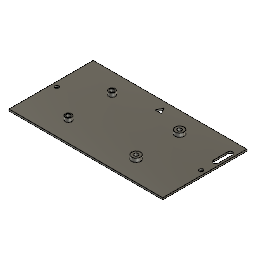
smmb_inner-middle (Autodesk Fusion 360 design; units mm, degrees)
Autodesk Fusion 360 part; units mm, degrees
sketch "Sketch1" plane through (0, 0, 0) normal (0, 0, 1) x (1, 0, 0)
  line L0 (0, 0) -> (127.5, 0)
  line L1 (127.5, 0) -> (127.5, 70)
  line L2 (127.5, 70) -> (0, 70)
  line L3 (0, 70) -> (0, 0)
  circle A0 centre (4, 35.763) radius 1.55
  line L4 (63.75, 0) -> (63.75, 70) construction
  circle A1 centre (123.5, 35.763) radius 1.55
  line L5 (66.25, 60) -> (61.25, 60)
  line L6 (61.25, 60) -> (61.25, 65)
  line L7 (61.25, 65) -> (66.25, 65)
  line L8 (66.25, 65) -> (66.25, 60)
  line L9 (66.25, 60) -> (61.25, 65) construction
  line L10 (61.25, 60) -> (66.25, 65) construction
  line L11 (63.75, 65) -> (61.25, 60)
  line L12 (63.75, 65) -> (66.25, 60)
  point P0 (63.75, 62.5)
  dimension "d1" = 127.5
  dimension "d2" = 70
  dimension "d3" = 3.1
  dimension "d4" = 35.763
  dimension "d5" = 4
  dimension "d8" = 5
  dimension "d9" = 5
  dimension "d12" = 5
  constraint horizontal L0
  constraint vertical L1
  constraint horizontal L2
  constraint vertical L3
  constraint coincident L0.start L3.end
  constraint midpoint L0 L4.start
  constraint midpoint L2 L4.end
  constraint symmetric A0 L4 A1
  constraint perpendicular L5 L6
  constraint parallel L5 L7
  constraint parallel L6 L8
  constraint horizontal L5
  constraint coincident L9 P0
  constraint coincident L10 P0
  constraint coincident L4 P0
  constraint midpoint L7 L11.start
  measures "d1" distance of L0.start L0.end
  measures "d2" distance of L0.start L2.end
  measures "d3" diameter of A0
  measures "d4" distance of L0 A0.centre
  measures "d5" distance of L3 A0.centre
  measures "d8" distance of L5.end L6.end
  measures "d9" distance of L6.end L7.end
  measures "d12" distance of L2 L7
extrude "Extrude1" add sketch "Sketch1" along normal blind 1.5 contours L0 L1 L2 L3 | L7 L8 L12 | L5 L11 L12 | L6 L7 L11
extrude "Extrude2" cut sketch "Sketch1" along normal blind 3 contours L5 L11 L12
sketch "Sketch2" plane through (0, 0, 1.5) normal (0, 0, 1) x (-1, 0, 0)
  line L0 (-63.75, -65) -> (-66.25, -60)
  line L1 (-66.25, -60) -> (-61.25, -60)
  line L2 (-61.25, -60) -> (-63.75, -65)
  circle A0 centre (-123.5, -35.763) radius 1.55
  circle A1 centre (-4, -35.763) radius 1.55
  line L3 (0, -70) -> (0, 0)
  line L4 (0, 0) -> (-127.5, 0)
  line L5 (-127.5, 0) -> (-127.5, -70)
  line L6 (-127.5, -70) -> (0, -70)
  line L7 (-90.5, -15) -> (-30.5, -15)
  line L8 (-30.5, -15) -> (-30.5, -55)
  line L9 (-30.5, -55) -> (-90.5, -55)
  line L10 (-90.5, -55) -> (-90.5, -15)
  line L11 (-90.5, -15) -> (-30.5, -55) construction
  line L12 (-30.5, -15) -> (-90.5, -55) construction
  circle A2 centre (-32.5, -53) radius 1.65
  circle A3 centre (-32.5, -53) radius 2.65
  circle A4 centre (-32.5, -17) radius 1.65
  circle A5 centre (-32.5, -17) radius 2.65
  circle A6 centre (-88.5, -53) radius 1.65
  circle A7 centre (-88.5, -53) radius 3.65
  circle A8 centre (-88.5, -17) radius 1.65
  circle A9 centre (-88.5, -17) radius 3.65
  line L13 (-123.5, -35.763) -> (-123.5, 0) construction
  line L14 (-123.5, -35.763) -> (-123.5, -70) construction
  line L15 (-125.5, -48) -> (-125.5, -60)
  arc A10 (-125.5, -60) -> (-121.5, -60) centre (-123.5, -60) ccw
  line L16 (-121.5, -60) -> (-121.5, -48)
  arc A11 (-121.5, -48) -> (-125.5, -48) centre (-123.5, -48) ccw
  line L17 (-123.5, -48) -> (-123.5, -60) construction
  point P0 (-60.5, -35)
  dimension "d13" = 40
  dimension "d14" = 60
  dimension "d15" = 15
  dimension "d16" = 37
  dimension "d17" = 3.3
  dimension "d18" = 5.3
  dimension "d19" = 2
  dimension "d20" = 2
  dimension "d21" = 3.3
  dimension "d22" = 5.3
  dimension "d23" = 2
  dimension "d24" = 2
  dimension "d25" = 3.3
  dimension "d26" = 7.3
  dimension "d27" = 2
  dimension "d28" = 2
  dimension "d29" = 3.3
  dimension "d30" = 7.3
  dimension "d31" = 2
  dimension "d32" = 2
  dimension "d37" = 4
  dimension "d38" = 10
  dimension "d39" = 12
  constraint perpendicular L7 L8
  constraint parallel L7 L9
  constraint parallel L8 L10
  constraint horizontal L7
  constraint coincident L11 P0
  constraint coincident L12 P0
  constraint concentric A2 A3
  constraint concentric A4 A5
  constraint concentric A6 A7
  constraint concentric A8 A9
  constraint coincident A0.centre L13.start
  constraint coincident L4 L13.end
  constraint perpendicular L4 L13
  constraint coincident L6 L14.end
  constraint perpendicular L6 L14
  constraint tangent L15 A10
  constraint tangent A10 L16
  constraint parallel L15 L16
  constraint tangent L16 A11
  constraint tangent L15 A11
  constraint parallel L14 L17
  constraint coincident L14 A11.centre
  measures "d13" distance of L7.end L8.end
  measures "d14" distance of L8.end L9.end
  measures "d15" distance of L4 L7
  measures "d16" distance of L5 L10
  measures "d17" diameter of A2
  measures "d18" diameter of A3
  measures "d19" distance of L9 A2.centre
  measures "d20" distance of L8 A2.centre
  measures "d21" diameter of A4
  measures "d22" diameter of A5
  measures "d23" distance of L8 A4.centre
  measures "d24" distance of L7 A4.centre
  measures "d25" diameter of A6
  measures "d26" diameter of A7
  measures "d27" distance of L9 A6.centre
  measures "d28" distance of L10 A6.centre
  measures "d29" diameter of A8
  measures "d30" diameter of A9
  measures "d31" distance of L10 A8.centre
  measures "d32" distance of L7 A8.centre
  measures "d37" diameter of A10
  measures "d38" distance of L6 A10.centre
  measures "d39" distance of A11.centre A10.centre
extrude "Extrude3" add sketch "Sketch2" along normal blind 3 contours L7 L10 A9 | L7 L10 A9 | L7 A5 | L7 L8 A5 | L9 L10 A7 | L9 L10 A7 | L8 A5 | L8 A3 | L8 L9 A3 | L9 A3 picked at (-32.5411, -15.1182) picked at (-32.5411, -54.8818)
extrude "Extrude4" cut sketch "Sketch2" against normal blind 4 contours A2 | A4 | A6 | A8
extrude "Extrude5" cut sketch "Sketch2" against normal blind 4 contours L15 A10 L16 A11
equation "d1 = 134 mm - 6 mm - 0.5 mm"
equation "d4 = 0.763 mm + 35 mm"
equation "d5 = 7 mm - 3 mm"
equation "d18 = d17 + 2 mm"
equation "d21 = d17"
equation "d22 = d18"
equation "d23 = d20"
equation "d24 = d19"
equation "d25 = d17"
equation "d26 = d25 + 4 mm"
equation "d27 = d19"
equation "d28 = d20"
equation "d29 = d25"
equation "d30 = d26"
equation "d31 = d28"
equation "d32 = d27"
